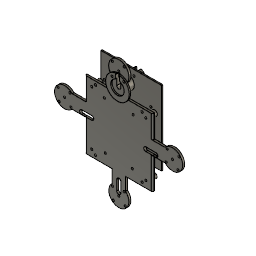
PX4-Jetson-GPS-Drone-Frame-v1 ✅ (Autodesk Fusion 360 design; units mm, degrees)
part number: 2026-08-23-16-08-48-525
Autodesk Fusion 360 part; units mm, degrees
note: some values were not read from the file. Chosen so that the rebuilt part matches the saved one: a direction.
sketch "Sketch1" plane through (0, 0, 0) normal (0, 1, 0) x (1, 0, 0)
  line L0 (50, -50) -> (-50, -50)
  line L1 (-50, -50) -> (-50, 50)
  line L2 (-50, 50) -> (50, 50)
  line L3 (50, 50) -> (50, -50)
  line L4 (50, -50) -> (-50, 50) construction
  line L5 (-50, -50) -> (50, 50) construction
  dimension "d1" = 100
  dimension "d2" = 100
  constraint horizontal L0
  constraint perpendicular L0 L1
  constraint parallel L0 L2
  constraint parallel L1 L3
  constraint coincident L4 origin
  constraint coincident L5 origin
  measures "d1" distance of L0.end L1.end
  measures "d2" distance of L1.end L2.end
extrude "Extrude1" add sketch "Sketch1" along normal blind 3
sketch "Sketch2" plane through (0, 0, 0) normal (0, 1, 0) x (1, 0, 0)
  line L0 (89.7731, -16.5642) -> (-90.2269, -16.5642)
  line L1 (-90.2269, -16.5642) -> (-90.2269, 3.4358)
  line L2 (-90.2269, 3.4358) -> (89.7731, 3.4358)
  line L3 (89.7731, 3.4358) -> (89.7731, -16.5642)
  line L4 (89.7731, -16.5642) -> (-90.2269, 3.4358) construction
  line L5 (-90.2269, -16.5642) -> (89.7731, 3.4358) construction
  line L6 (-10, -90) -> (10, -90)
  line L7 (10, -90) -> (10, 90)
  line L8 (10, 90) -> (-10, 90)
  line L9 (-10, 90) -> (-10, -90)
  line L10 (-10, -90) -> (10, 90) construction
  line L11 (10, -90) -> (-10, 90) construction
  point P0 (-0.2269, -6.5642)
  dimension "d9" = 180
  dimension "d10" = 20
  dimension "d11" = 20
  dimension "d12" = 180
  constraint horizontal L0
  constraint perpendicular L0 L1
  constraint parallel L0 L2
  constraint parallel L1 L3
  constraint coincident L4 P0
  constraint coincident L5 P0
  constraint horizontal L6
  constraint perpendicular L6 L7
  constraint parallel L6 L8
  constraint parallel L7 L9
  constraint coincident L10 origin
  constraint coincident L11 origin
  measures "d9" distance of L1.end L2.end
  measures "d10" distance of L0.start L2.end
  measures "d11" distance of L7.end L8.end
  measures "d12" distance of L6.start L8.end
extrude "Extrude2" add sketch "Sketch2" along normal blind 3
sketch "Sketch3" plane through (0, 0, 0) normal (0, -1, 0) x (1, 0, 0)
  line L0 (-10, 50) -> (-50, 50)
  line L1 (-50, 50) -> (-50, 16.5642)
  line L2 (-50, 16.5642) -> (-90.2269, 16.5642)
  line L3 (-90.2269, 16.5642) -> (-90.2269, -3.4358)
  line L4 (-90.2269, -3.4358) -> (-50, -3.4358)
  line L5 (-50, -3.4358) -> (-50, -50)
  line L6 (-50, -50) -> (-10, -50)
  line L7 (-10, -50) -> (-10, -90)
  line L8 (-10, -90) -> (10, -90)
  line L9 (10, -90) -> (10, -50)
  line L10 (10, -50) -> (50, -50)
  line L11 (50, -50) -> (50, -3.4358)
  line L12 (50, -3.4358) -> (89.7731, -3.4358)
  line L13 (89.7731, -3.4358) -> (89.7731, 16.5642)
  line L14 (89.7731, 16.5642) -> (50, 16.5642)
  line L15 (50, 16.5642) -> (50, 50)
  line L16 (50, 50) -> (10, 50)
  line L17 (10, 50) -> (10, 90)
  line L18 (10, 90) -> (-10, 90)
  line L19 (-10, 90) -> (-10, 50)
  circle A0 centre (79.7731, 6.5642) radius 1.5
  circle A1 centre (-80.2269, 6.5642) radius 1.5
  circle A2 centre (0, 80) radius 1.5
  circle A3 centre (0, -80) radius 1.5
  dimension "d15" = 3
  dimension "d16" = 10
  dimension "d17" = 10
  dimension "d18" = 3
  dimension "d19" = 10
  dimension "d20" = 10
  dimension "d21" = 3
  dimension "d22" = 10
  dimension "d23" = 10
  dimension "d24" = 3
  dimension "d25" = 10
  dimension "d26" = 10
  measures "d15" diameter of A0
  measures "d16" distance of L13 A0.centre
  measures "d17" distance of L12 A0.centre
  measures "d18" diameter of A1
  measures "d19" distance of L3 A1.centre
  measures "d20" distance of L4 A1.centre
  measures "d21" diameter of A2
  measures "d22" distance of L18 A2.centre
  measures "d23" distance of L19 A2.centre
  measures "d24" diameter of A3
  measures "d25" distance of L7 A3.centre
  measures "d26" distance of L8 A3.centre
extrude "Extrude3" cut sketch "Sketch3" against normal through all contours A0 | A1 | A2 | A3
sketch "Sketch4" plane through (0, 0, 0) normal (0, 1, 0) x (1, 0, 0)
  circle A0 centre (79.5401, -6.6988) radius 15
  dimension "d28" = 30
  measures "d28" diameter of A0
sketch "Sketch5" plane through (0, 0, 0) normal (0, 1, 0) x (1, 0, 0)
extrude "Extrude4" add sketch "Sketch4" along normal blind 3
sketch "Sketch6" plane through (0, 0, 0) normal (0, 1, 0) x (1, 0, 0)
  circle A0 centre (0, -80) radius 15
  dimension "d31" = 30
  measures "d31" diameter of A0
extrude "Extrude5" add sketch "Sketch6" along normal blind 3
sketch "Sketch7" plane through (0, 0, 0) normal (0, 1, 0) x (1, 0, 0)
  circle A0 centre (-80.2727, -6.5181) radius 15
  dimension "d34" = 30
  measures "d34" diameter of A0
extrude "Extrude6" add sketch "Sketch7" along normal blind 3
sketch "Sketch8" plane through (0, 0, 0) normal (0, 1, 0) x (1, 0, 0)
  circle A0 centre (0, 80) radius 15
  dimension "d37" = 30
  measures "d37" diameter of A0
extrude "Extrude7" add sketch "Sketch8" along normal blind 3
sketch "Sketch9" plane through (0, 0, 0) normal (0, -1, 0) x (1, 0, 0)
  arc A0 (-10, -68.8197) -> (10, -68.8197) centre (0, -80) ccw
  line L0 (10, -68.8197) -> (10, -50)
  line L1 (10, -50) -> (50, -50)
  line L2 (50, -50) -> (50, -3.4358)
  line L3 (50, -3.4358) -> (68.4816, -3.4358)
  arc A1 (68.4816, -3.4358) -> (68.2409, 16.5642) centre (79.5401, 6.6988) ccw
  line L4 (68.2409, 16.5642) -> (50, 16.5642)
  line L5 (50, 16.5642) -> (50, 50)
  line L6 (50, 50) -> (10, 50)
  line L7 (10, 50) -> (10, 68.8197)
  arc A2 (10, 68.8197) -> (-10, 68.8197) centre (0, 80) ccw
  line L8 (-10, 68.8197) -> (-10, 50)
  line L9 (-10, 50) -> (-50, 50)
  line L10 (-50, 50) -> (-50, 16.5642)
  line L11 (-50, 16.5642) -> (-69.1338, 16.5642)
  arc A3 (-69.1338, 16.5642) -> (-69.0513, -3.4358) centre (-80.2727, 6.5181) ccw
  line L12 (-69.0513, -3.4358) -> (-50, -3.4358)
  line L13 (-50, -3.4358) -> (-50, -50)
  line L14 (-50, -50) -> (-10, -50)
  line L15 (-10, -50) -> (-10, -68.8197)
  circle A4 centre (79.5401, 6.6988) radius 1.5
  circle A5 centre (-80.2727, 6.5181) radius 1.5
  circle A6 centre (0, -80) radius 1.5
  circle A7 centre (0, 80) radius 1.5
  dimension "d40" = 3
  dimension "d41" = 3
  dimension "d42" = 3
  dimension "d43" = 3
  constraint concentric A1 A4
  constraint concentric A3 A5
  constraint concentric A0 A6
  constraint concentric A2 A7
  measures "d40" diameter of A4
  measures "d41" diameter of A5
  measures "d42" diameter of A6
  measures "d43" diameter of A7
extrude "Extrude8" cut sketch "Sketch9" against normal through all contours A4 | A5 | A6 | A7
sketch "Sketch10" plane through (0, 0, 50) normal (0, 0, 1) x (-1, 0, 0)
  line L0 (-10, -3) -> (-10, 0)
  line L1 (-10, 0) -> (-50, 0)
  line L2 (-50, 0) -> (-50, -3)
  line L3 (-50, -3) -> (-10, -3)
sketch "Sketch11" plane through (0, 0, 0) normal (0, -1, 0) x (1, 0, 0)
  circle A0 centre (-80.2727, 6.5181) radius 1.5
  circle A1 centre (79.5401, 6.6988) radius 1.5
  circle A2 centre (0, 80) radius 1.5
  circle A3 centre (0, -80) radius 1.5
  arc A4 (-10, -68.8197) -> (10, -68.8197) centre (0, -80) ccw
  line L0 (10, -68.8197) -> (10, -50)
  line L1 (10, -50) -> (50, -50)
  line L2 (50, -50) -> (50, -3.4358)
  line L3 (50, -3.4358) -> (68.4816, -3.4358)
  arc A5 (68.4816, -3.4358) -> (68.2409, 16.5642) centre (79.5401, 6.6988) ccw
  line L4 (68.2409, 16.5642) -> (50, 16.5642)
  line L5 (50, 16.5642) -> (50, 50)
  line L6 (50, 50) -> (10, 50)
  line L7 (10, 50) -> (10, 68.8197)
  arc A6 (10, 68.8197) -> (-10, 68.8197) centre (0, 80) ccw
  line L8 (-10, 68.8197) -> (-10, 50)
  line L9 (-10, 50) -> (-50, 50)
  line L10 (-50, 50) -> (-50, 16.5642)
  line L11 (-50, 16.5642) -> (-69.1338, 16.5642)
  arc A7 (-69.1338, 16.5642) -> (-69.0513, -3.4358) centre (-80.2727, 6.5181) ccw
  line L12 (-69.0513, -3.4358) -> (-50, -3.4358)
  line L13 (-50, -3.4358) -> (-50, -50)
  line L14 (-50, -50) -> (-10, -50)
  line L15 (-10, -50) -> (-10, -68.8197)
  circle A8 centre (40, 40) radius 1.5
  circle A9 centre (-40, 40) radius 1.5
  circle A10 centre (40, -40) radius 1.5
  circle A11 centre (-40, -40) radius 1.5
  dimension "d45" = 3
  dimension "d46" = 10
  dimension "d47" = 10
  dimension "d48" = 3
  dimension "d49" = 10
  dimension "d50" = 10
  dimension "d51" = 3
  dimension "d52" = 10
  dimension "d53" = 10
  dimension "d54" = 3
  dimension "d55" = 10
  measures "d45" diameter of A8
  measures "d46" distance of L6 A8.centre
  measures "d47" distance of L5 A8.centre
  measures "d48" diameter of A9
  measures "d49" distance of L10 A9.centre
  measures "d50" distance of L9 A9.centre
  measures "d51" diameter of A10
  measures "d52" distance of L2 A10.centre
  measures "d53" distance of L1 A10.centre
  measures "d54" diameter of A11
  measures "d55" distance of L14 A11.centre
extrude "Extrude9" cut sketch "Sketch11" against normal through all contours A8 | A9 | A10 | A11
sketch "Sketch12" plane through (0, 3, 0) normal (0, 1, 0) x (-1, 0, 0)
  line L0 (10, -68.8197) -> (10, -50)
  line L1 (10, -50) -> (50, -50)
  line L2 (50, -50) -> (50, -3.4358)
  line L3 (50, -3.4358) -> (69.0513, -3.4358)
  arc A0 (69.0513, -3.4358) -> (69.1338, 16.5642) centre (80.2727, 6.5181) ccw
  line L4 (69.1338, 16.5642) -> (50, 16.5642)
  line L5 (50, 16.5642) -> (50, 50)
  line L6 (50, 50) -> (10, 50)
  line L7 (10, 50) -> (10, 68.8197)
  arc A1 (10, 68.8197) -> (-10, 68.8197) centre (0, 80) ccw
  line L8 (-10, 68.8197) -> (-10, 50)
  line L9 (-10, 50) -> (-50, 50)
  line L10 (-50, 50) -> (-50, 16.5642)
  line L11 (-50, 16.5642) -> (-68.2409, 16.5642)
  arc A2 (-68.2409, 16.5642) -> (-68.4816, -3.4358) centre (-79.5401, 6.6988) ccw
  line L12 (-68.4816, -3.4358) -> (-50, -3.4358)
  line L13 (-50, -3.4358) -> (-50, -50)
  line L14 (-50, -50) -> (-10, -50)
  line L15 (-10, -50) -> (-10, -68.8197)
  arc A3 (-10, -68.8197) -> (10, -68.8197) centre (0, -80) ccw
  circle A4 centre (0, -80) radius 1.5
  circle A5 centre (0, 80) radius 1.5
  circle A6 centre (-79.5401, 6.6988) radius 1.5
  circle A7 centre (80.2727, 6.5181) radius 1.5
  circle A8 centre (40, -40) radius 1.5
  circle A9 centre (40, 40) radius 1.5
  circle A10 centre (-40, -40) radius 1.5
  circle A11 centre (-40, 40) radius 1.5
  line L16 (-22, -42) -> (22, -42)
  line L17 (22, -42) -> (22, 42)
  line L18 (22, 42) -> (-22, 42)
  line L19 (-22, 42) -> (-22, -42)
  line L20 (-22, -42) -> (22, 42) construction
  line L21 (22, -42) -> (-22, 42) construction
  dimension "d57" = 44
  dimension "d58" = 84
  constraint horizontal L16
  constraint perpendicular L16 L17
  constraint parallel L16 L18
  constraint parallel L17 L19
  constraint coincident L20 origin
  constraint coincident L21 origin
  measures "d57" distance of L16.start L16.end
  measures "d58" distance of L16.end L17.end
sketch "Sketch13" plane through (0, 3, 0) normal (0, 1, 0) x (-1, 0, 0)
  line L0 (-39.5, -50) -> (39.5, -50)
  line L1 (39.5, -50) -> (39.5, 50)
  line L2 (39.5, 50) -> (-39.5, 50)
  line L3 (-39.5, 50) -> (-39.5, -50)
  line L4 (-39.5, -50) -> (39.5, 50) construction
  line L5 (39.5, -50) -> (-39.5, 50) construction
  dimension "d59" = 100
  dimension "d60" = 79
  constraint horizontal L0
  constraint perpendicular L0 L1
  constraint parallel L0 L2
  constraint parallel L1 L3
  constraint coincident L4 origin
  constraint coincident L5 origin
  measures "d59" distance of L0.end L1.end
  measures "d60" distance of L0.start L0.end
sketch "Sketch14" plane through (0, 3, 0) normal (0, 1, 0) x (-1, 0, 0)
sketch "Sketch15" plane through (0, 3, 0) normal (0, 1, 0) x (-1, 0, 0)
  circle A0 centre (40, -40) radius 4
  circle A1 centre (-40, -40) radius 4
  circle A2 centre (-40, 40) radius 4
  circle A3 centre (40, 40) radius 4
  dimension "d61" = 8
  dimension "d62" = 8
  dimension "d63" = 8
  dimension "d64" = 8
  measures "d61" diameter of A0
  measures "d62" diameter of A1
  measures "d63" diameter of A2
  measures "d64" diameter of A3
extrude "Extrude10" add sketch "Sketch15" along normal blind 10
sketch "Sketch16" plane through (0, 3, 0) normal (0, 1, 0) x (-1, 0, 0)
  circle A0 centre (-40, -40) radius 1.5
  circle A1 centre (40, -40) radius 1.5
  circle A2 centre (40, 40) radius 1.5
  circle A3 centre (-40, 40) radius 1.5
  dimension "d67" = 3
  dimension "d68" = 3
  dimension "d69" = 3
  dimension "d70" = 3
  measures "d67" diameter of A0
  measures "d68" diameter of A1
  measures "d69" diameter of A2
  measures "d70" diameter of A3
sketch "Sketch17" plane through (0, 13, 0) normal (0, 1, 0) x (-1, 0, 0)
  circle A0 centre (-40, -40) radius 4
  line L0 (-50.2773, -29.6179) -> (39.7227, -29.6179)
  line L1 (39.7227, -29.6179) -> (39.7227, 80.3821)
  line L2 (39.7227, 80.3821) -> (-50.2773, 80.3821)
  line L3 (-50.2773, 80.3821) -> (-50.2773, -29.6179)
  line L4 (-50.2773, -29.6179) -> (39.7227, 80.3821) construction
  line L5 (39.7227, -29.6179) -> (-50.2773, 80.3821) construction
  point P0 (-5.2773, 25.3821)
  dimension "d71" = 90
  dimension "d72" = 110
  constraint horizontal L0
  constraint perpendicular L0 L1
  constraint parallel L0 L2
  constraint parallel L1 L3
  constraint coincident L4 P0
  constraint coincident L5 P0
  measures "d71" distance of L0.start L0.end
  measures "d72" distance of L0.end L1.end
extrude "Extrude11" add sketch "Sketch17" along normal blind 2 contours L0 L1 L2 L3
sketch "Sketch18" plane through (0, 0, 0) normal (0, -1, 0) x (1, 0, 0)
  arc A0 (-10, -68.8197) -> (10, -68.8197) centre (0, -80) ccw
  line L0 (10, -68.8197) -> (10, -50)
  line L1 (10, -50) -> (50, -50)
  line L2 (50, -50) -> (50, -3.4358)
  line L3 (50, -3.4358) -> (68.4816, -3.4358)
  arc A1 (68.4816, -3.4358) -> (68.2409, 16.5642) centre (79.5401, 6.6988) ccw
  line L4 (68.2409, 16.5642) -> (50, 16.5642)
  line L5 (50, 16.5642) -> (50, 50)
  line L6 (50, 50) -> (10, 50)
  line L7 (10, 50) -> (10, 68.8197)
  arc A2 (10, 68.8197) -> (-10, 68.8197) centre (0, 80) ccw
  line L8 (-10, 68.8197) -> (-10, 50)
  line L9 (-10, 50) -> (-50, 50)
  line L10 (-50, 50) -> (-50, 16.5642)
  line L11 (-50, 16.5642) -> (-69.1338, 16.5642)
  arc A3 (-69.1338, 16.5642) -> (-69.0513, -3.4358) centre (-80.2727, 6.5181) ccw
  line L12 (-69.0513, -3.4358) -> (-50, -3.4358)
  line L13 (-50, -3.4358) -> (-50, -50)
  line L14 (-50, -50) -> (-10, -50)
  line L15 (-10, -50) -> (-10, -68.8197)
  circle A4 centre (0, -80) radius 1.5
  circle A5 centre (0, 80) radius 1.5
  circle A6 centre (79.5401, 6.6988) radius 1.5
  circle A7 centre (-80.2727, 6.5181) radius 1.5
  circle A8 centre (-40, -40) radius 1.5
  circle A9 centre (-40, 40) radius 1.5
  circle A10 centre (40, -40) radius 1.5
  circle A11 centre (40, 40) radius 1.5
  line L16 (-22, -42.4) -> (22, -42.4)
  line L17 (22, -42.4) -> (22, 42.4)
  line L18 (22, 42.4) -> (-22, 42.4)
  line L19 (-22, 42.4) -> (-22, -42.4)
  line L20 (-22, -42.4) -> (22, 42.4) construction
  line L21 (22, -42.4) -> (-22, 42.4) construction
  dimension "d75" = 44
  dimension "d76" = 84.8
  constraint horizontal L16
  constraint perpendicular L16 L17
  constraint parallel L16 L18
  constraint parallel L17 L19
  constraint coincident L20 origin
  constraint coincident L21 origin
  measures "d75" distance of L16.start L16.end
  measures "d76" distance of L16.end L17.end
sketch "Sketch19" plane through (0, 0, 0) normal (0, -1, 0) x (1, 0, 0)
extrude "Extrude12" cut sketch "Sketch18" against normal through all contours A8 | A9 | A10 | A11
sketch "Sketch20" plane through (0, 0, 0) normal (0, -1, 0) x (1, 0, 0)
  arc A0 (-10, -68.8197) -> (10, -68.8197) centre (0, -80) ccw
  line L0 (10, -68.8197) -> (10, -50)
  line L1 (10, -50) -> (50, -50)
  line L2 (50, -50) -> (50, -3.4358)
  line L3 (50, -3.4358) -> (68.4816, -3.4358)
  arc A1 (68.4816, -3.4358) -> (68.2409, 16.5642) centre (79.5401, 6.6988) ccw
  line L4 (68.2409, 16.5642) -> (50, 16.5642)
  line L5 (50, 16.5642) -> (50, 50)
  line L6 (50, 50) -> (10, 50)
  line L7 (10, 50) -> (10, 68.8197)
  arc A2 (10, 68.8197) -> (-10, 68.8197) centre (0, 80) ccw
  line L8 (-10, 68.8197) -> (-10, 50)
  line L9 (-10, 50) -> (-50, 50)
  line L10 (-50, 50) -> (-50, 16.5642)
  line L11 (-50, 16.5642) -> (-69.1338, 16.5642)
  arc A3 (-69.1338, 16.5642) -> (-69.0513, -3.4358) centre (-80.2727, 6.5181) ccw
  line L12 (-69.0513, -3.4358) -> (-50, -3.4358)
  line L13 (-50, -3.4358) -> (-50, -50)
  line L14 (-50, -50) -> (-10, -50)
  line L15 (-10, -50) -> (-10, -68.8197)
  circle A4 centre (0, -80) radius 1.5
  circle A5 centre (0, 80) radius 1.5
  circle A6 centre (79.5401, 6.6988) radius 1.5
  circle A7 centre (-80.2727, 6.5181) radius 1.5
  circle A8 centre (-40, -40) radius 1.5
  circle A9 centre (-40, 40) radius 1.5
  circle A10 centre (40, -40) radius 1.5
  circle A11 centre (40, 40) radius 1.5
  line L16 (39.5, 50) -> (-39.5, 50)
  line L17 (-39.5, 50) -> (-39.5, -50)
  line L18 (-39.5, -50) -> (39.5, -50)
  line L19 (39.5, -50) -> (39.5, 50)
  line L20 (39.5, 50) -> (-39.5, -50) construction
  line L21 (-39.5, 50) -> (39.5, -50) construction
  dimension "d78" = 79
  dimension "d79" = 100
  constraint horizontal L16
  constraint perpendicular L16 L17
  constraint parallel L16 L18
  constraint parallel L17 L19
  constraint coincident L20 origin
  constraint coincident L21 origin
  measures "d78" distance of L16.start L16.end
  measures "d79" distance of L16.end L17.end
sketch "Sketch21" plane through (0, 0, 0) normal (0, -1, 0) x (1, 0, 0)
  circle A0 centre (34.5, 45) radius 1.6
  line L0 (39.5, -50) -> (39.5, 50)
  line L1 (39.5, 50) -> (-39.5, 50)
  circle A1 centre (-34.5, 45) radius 1.6
  line L2 (-39.5, 50) -> (-39.5, -50)
  circle A2 centre (34.5, -45) radius 1.6
  line L3 (-39.5, -50) -> (39.5, -50)
  circle A3 centre (-34.5, -45) radius 1.6
  point P0 (-39.5, 50)
  point P1 (39.5, 50)
  point P2 (39.5, -50)
  point P3 (-39.5, -50)
  dimension "d80" = 3.2
  dimension "d81" = 5
  dimension "d82" = 5
  dimension "d83" = 3.2
  dimension "d84" = 5
  dimension "d85" = 5
  dimension "d86" = 3.2
  dimension "d87" = 5
  dimension "d88" = 5
  dimension "d89" = 3.2
  dimension "d90" = 5
  dimension "d91" = 5
  measures "d80" diameter of A0
  measures "d81" distance of A0.centre L0
  measures "d82" distance of A0.centre L1
  measures "d83" diameter of A1
  measures "d84" distance of A1.centre L2
  measures "d85" distance of L1 A1.centre
  measures "d86" diameter of A2
  measures "d87" distance of L0 A2.centre
  measures "d88" distance of A2.centre L3
  measures "d89" diameter of A3
  measures "d90" distance of L2 A3.centre
  measures "d91" distance of L3 A3.centre
extrude "Extrude13" cut sketch "Sketch21" against normal through all contours A0 | A1 | A2 | A3
sketch "Sketch22" plane through (0, 0, 0) normal (0, 1, 0) x (1, 0, 0)
  line L0 (-19.9597, -27.3903) -> (19.9597, 27.3903) construction
  line L1 (19.9597, -27.3903) -> (-19.9597, 27.3903) construction
  constraint coincident L0 origin
  constraint coincident L1 origin
sketch "Sketch23" plane through (0, 0, 0) normal (0, 1, 0) x (1, 0, 0)
  circle A0 centre (0, -60) radius 10
  dimension "d93" = 20
  measures "d93" diameter of A0
extrude "Extrude14" add sketch "Sketch23" along normal blind 30
sketch "Sketch24" plane through (0, 0, 0) normal (0, -1, 0) x (1, 0, 0)
sketch "Sketch25" plane through (0, 0, 0) normal (0, -1, 0) x (1, 0, 0)
  circle A0 centre (0, 60) radius 10
  circle A1 centre (0, 60) radius 17.5
  dimension "d97" = 20
  dimension "d98" = 35
  constraint concentric A0 A1
  measures "d97" diameter of A0
  measures "d98" diameter of A1
extrude "Extrude15" add sketch "Sketch25" along normal blind 2
sketch "Sketch26" plane through (0, -2, 0) normal (0, -1, 0) x (1, 0, 0)
  circle A0 centre (0, 60) radius 10
  circle A1 centre (0, 60) radius 17.5
sketch "Sketch27" plane through (0, 0, 0) normal (0, 1, 0) x (1, 0, 0)
  circle A0 centre (79.5185, -6.7286) radius 1.6
  line L0 (40, -3) -> (55, -3)
  arc A1 (55, -3) -> (55, 3) centre (55, 0) ccw
  line L1 (55, 3) -> (40, 3)
  arc A2 (40, 3) -> (40, -3) centre (40, 0) ccw
  line L2 (40, 0) -> (55, 0) construction
  dimension "d101" = 3.2
  dimension "d102" = 6
  dimension "d103" = 15
  constraint tangent L0 A1
  constraint tangent A1 L1
  constraint parallel L0 L1
  constraint tangent L1 A2
  constraint tangent L0 A2
  constraint horizontal L2
  measures "d101" diameter of A0
  measures "d102" diameter of A1
  measures "d103" distance of A2.centre A1.centre
extrude "Extrude16" cut sketch "Sketch27" along normal through all contours L0 A1 L1 A2
sketch "Sketch28" plane through (0, 0, 0) normal (0, 1, 0) x (1, 0, 0)
  line L0 (-40, 3) -> (-55, 3)
  arc A0 (-55, 3) -> (-55, -3) centre (-55, 0) ccw
  line L1 (-55, -3) -> (-40, -3)
  arc A1 (-40, -3) -> (-40, 3) centre (-40, 0) ccw
  line L2 (-40, 0) -> (-55, 0) construction
  dimension "d105" = 6
  dimension "d106" = 15
  constraint tangent L0 A0
  constraint tangent A0 L1
  constraint parallel L0 L1
  constraint tangent L1 A1
  constraint tangent L0 A1
  constraint horizontal L2
  measures "d105" diameter of A0
  measures "d106" distance of A1.centre A0.centre
extrude "Extrude17" cut sketch "Sketch28" along normal through all
sketch "Sketch29" plane through (0, -2, 0) normal (0, -1, 0) x (1, 0, 0)
  line L0 (3, 60) -> (3, 75)
  arc A0 (3, 75) -> (-3, 75) centre (0, 75) ccw
  line L1 (-3, 75) -> (-3, 60)
  arc A1 (-3, 60) -> (3, 60) centre (0, 60) ccw
  line L2 (0, 60) -> (0, 75) construction
  line L3 (-3, -60) -> (-3, -75)
  arc A2 (-3, -75) -> (3, -75) centre (0, -75) ccw
  line L4 (3, -75) -> (3, -60)
  arc A3 (3, -60) -> (-3, -60) centre (0, -60) ccw
  line L5 (0, -60) -> (0, -75) construction
  dimension "d108" = 6
  dimension "d109" = 15
  dimension "d110" = 6
  dimension "d111" = 15
  constraint tangent L0 A0
  constraint tangent A0 L1
  constraint parallel L0 L1
  constraint tangent L1 A1
  constraint tangent L0 A1
  constraint vertical L2
  constraint tangent L3 A2
  constraint tangent A2 L4
  constraint parallel L3 L4
  constraint tangent L4 A3
  constraint tangent L3 A3
  constraint vertical L5
  measures "d108" diameter of A0
  measures "d109" distance of A1.centre A0.centre
  measures "d110" diameter of A2
  measures "d111" distance of A3.centre A2.centre
extrude "Extrude18" cut sketch "Sketch29" against normal through all
sketch "Sketch30" plane through (0, 0, 0) normal (0, -1, 0) x (1, 0, 0)
sketch "Sketch31" plane through (0, 3, 0) normal (0, 1, 0) x (-1, 0, 0)
fillet "Fillet1" radius 2 4 edges at (50, 0, 33.2821) (50, 0, -26.7179) (-50, 0, -26.7179) (-50, 0, 33.2821)
sketch "Sketch32" plane through (0, 0, 0) normal (0, -1, 0) x (1, 0, 0)
  circle A0 centre (70.0401, -1.3012) radius 1.5
  circle A1 centre (87.5401, -2.8012) radius 1.5
  circle A2 centre (89.0401, 14.6988) radius 1.5
  circle A3 centre (71.5401, 16.1988) radius 1.5
  point P0 (79.5401, 6.6988)
  dimension "d115" = 3
  dimension "d116" = 9.5
  dimension "d117" = 8
  dimension "d119" = 360
  measures "d115" diameter of A0
  measures "d116" horizontal distance of A0.centre P0
  measures "d117" vertical distance of A0.centre P0
extrude "Extrude19" cut sketch "Sketch32" against normal through all
sketch "Sketch33" plane through (0, 0, 0) normal (0, -1, 0) x (1, 0, 0)
  circle A0 centre (-70.7727, -1.4819) radius 1.5
  circle A1 centre (-89.7727, 14.5181) radius 1.5
  circle A2 centre (-72.2727, 16.0181) radius 1.5
  circle A3 centre (-88.2727, -2.9819) radius 1.5
  point P0 (-80.2727, 6.5181)
  point P1 (-72.2727, 16.0181)
  point P2 (-89.7727, 14.5181)
  point P3 (-88.2727, -2.9819)
  dimension "d121" = 3
  dimension "d122" = 9.5
  dimension "d123" = 8
  dimension "d125" = 360
  dimension "d126" = 3
  dimension "d127" = 3
  dimension "d128" = 3
  constraint coincident P2 A1.centre
  constraint coincident P1 A2.centre
  constraint coincident P3 A3.centre
  measures "d121" diameter of A0
  measures "d122" horizontal distance of A0.centre P0
  measures "d123" vertical distance of A0.centre P0
  measures "d126" diameter of A1
  measures "d127" diameter of A2
  measures "d128" diameter of A3
extrude "Extrude20" cut sketch "Sketch33" against normal through all
sketch "Sketch34" plane through (0, -2, 0) normal (0, -1, 0) x (1, 0, 0)
  circle A0 centre (9.5, 72) radius 1.5
  circle A1 centre (-8, 70.5) radius 1.5
  circle A2 centre (-9.5, 88) radius 1.5
  circle A3 centre (8, 89.5) radius 1.5
  point P0 (0, 80)
  point P1 (8, 89.5)
  point P2 (-9.5, 88)
  point P3 (-8, 70.5)
  dimension "d130" = 3
  dimension "d131" = 8
  dimension "d132" = 9.5
  dimension "d134" = 360
  dimension "d135" = 3
  dimension "d136" = 3
  dimension "d137" = 3
  constraint coincident P3 A1.centre
  constraint coincident P2 A2.centre
  constraint coincident P1 A3.centre
  measures "d130" diameter of A0
  measures "d131" vertical distance of A0.centre P0
  measures "d132" horizontal distance of A0.centre P0
  measures "d135" diameter of A1
  measures "d136" diameter of A2
  measures "d137" diameter of A3
extrude "Extrude21" cut sketch "Sketch34" against normal through all
sketch "Sketch35" plane through (0, 0, 0) normal (0, -1, 0) x (1, 0, 0)
  circle A0 centre (9.5, -88) radius 1.5
  circle A1 centre (-9.5, -72) radius 1.5
  circle A2 centre (8, -70.5) radius 1.5
  circle A3 centre (-8, -89.5) radius 1.5
  point P0 (0, -80)
  point P1 (8, -70.5)
  point P2 (-9.5, -72)
  point P3 (-8, -89.5)
  dimension "d139" = 3
  dimension "d140" = 8
  dimension "d141" = 9.5
  dimension "d143" = 360
  dimension "d144" = 3
  dimension "d145" = 3
  dimension "d146" = 3
  constraint coincident P2 A1.centre
  constraint coincident P1 A2.centre
  constraint coincident P3 A3.centre
  measures "d139" diameter of A0
  measures "d140" vertical distance of A0.centre P0
  measures "d141" horizontal distance of A0.centre P0
  measures "d144" diameter of A1
  measures "d145" diameter of A2
  measures "d146" diameter of A3
extrude "Extrude22" cut sketch "Sketch35" against normal through all
sketch "Sketch36" plane through (0, 0, 0) normal (0, -1, 0) x (1, 0, 0)
  line L0 (25, 40) -> (-25, 40)
  line L1 (-25, 40) -> (-25, -40)
  line L2 (-25, -40) -> (25, -40)
  line L3 (25, -40) -> (25, 40)
  line L4 (25, 40) -> (-25, -40) construction
  line L5 (-25, 40) -> (25, -40) construction
  dimension "d148" = 50
  dimension "d149" = 80
  constraint horizontal L0
  constraint perpendicular L0 L1
  constraint parallel L0 L2
  constraint parallel L1 L3
  constraint coincident L4 origin
  constraint coincident L5 origin
  measures "d148" distance of L0.start L0.end
  measures "d149" distance of L0.start L2.end
sketch "Sketch37" plane through (0, 0, 0) normal (0, -1, 0) x (1, 0, 0)
  circle A0 centre (21.278, 35) radius 1.5
  line L0 (39.5, 50) -> (-39.5, -50)
  line L1 (25, 40) -> (-25, 40)
  circle A1 centre (-21.278, 35) radius 1.5
  line L2 (-39.5, 50) -> (39.5, -50)
  circle A2 centre (20, -35) radius 1.5
  line L3 (25, -40) -> (25, 40)
  line L4 (-25, -40) -> (25, -40)
  circle A3 centre (-20, -35) radius 1.5
  line L5 (-25, 40) -> (-25, -40)
  dimension "d150" = 3
  dimension "d151" = 5
  dimension "d152" = 5
  dimension "d153" = 3
  dimension "d154" = 5
  dimension "d155" = 5
  dimension "d156" = 3
  dimension "d157" = 5
  dimension "d158" = 5
  dimension "d159" = 3
  dimension "d160" = 5
  dimension "d161" = 5
  measures "d150" diameter of A0
  measures "d151" distance of A0.centre L0
  measures "d152" distance of A0.centre L1
  measures "d153" diameter of A1
  measures "d154" distance of A1.centre L2
  measures "d155" distance of L1 A1.centre
  measures "d156" diameter of A2
  measures "d157" distance of A2.centre L3
  measures "d158" distance of A2.centre L4
  measures "d159" diameter of A3
  measures "d160" distance of A3.centre L5
  measures "d161" distance of L4 A3.centre
extrude "Extrude23" cut sketch "Sketch37" against normal through all contours A0 | A1 | A2 | A3
